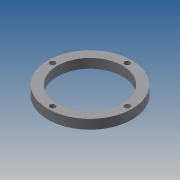
# Autodesk Inventor part: ring
Saved by Autodesk Inventor 2013 (Build 170138000, 138)
## iProperties
Created: 2017-03-30
Part Number: ring
Material: Generic
Document SubType Name: Modeling
Designer: employee
Density: 1 g/cm^3
Author: employee
Autodesk Inventor part; units mm, degrees
ref_plane "YZ Plane" through (0, 0, 0) normal (1, 0, 0) x (0, 1, 0)
ref_plane "XZ Plane" through (0, 0, 0) normal (0, 1, 0) x (-1, 0, 0)
ref_plane "XY Plane" through (0, 0, 0) normal (0, 0, 1) x (1, 0, 0)
sketch "Sketch1" plane through (0, 0, 0) normal (0, 0, 1) x (1, 0, 0)
  circle A0 centre (0, 0) radius 45
  circle A1 centre (0, 0) radius 35
  dimension "d0" = 70
  dimension "d2" = 90
  constraints: 2 centre point, 1 coincident
  measures "d0" diameter of A1
  measures "d2" diameter of A0
extrude "Extrusion1" add sketch "Sketch1" along normal blind 10
sketch "Sketch2" plane through (0, 0, 10) normal (0, 0, 1) x (1, 0, 0)
  circle A0 centre (0, 0) radius 35 projected
  circle A1 centre (0, 40) radius 1.75
  dimension "d5" = 40
  dimension "d6" = 3.5
  constraints: 1 centre point, 1 vertical alignment
  measures "d5" distance of A1.centre A0.centre
  measures "d6" diameter of A1
extrude "Extrusion2" cut sketch "Sketch2" against normal through all contours A1
sketch "Sketch3" plane through (0, 0, 10) normal (0, 0, 1) x (1, 0, 0)
  circle A0 centre (0, 40) radius 1.75 projected
  line L0 (3.1754, 40) -> (1.5877, 37.25)
  line L1 (1.5877, 37.25) -> (-1.5877, 37.25)
  line L2 (-1.5877, 37.25) -> (-3.1754, 40)
  line L3 (-3.1754, 40) -> (-1.5877, 42.75)
  line L4 (-1.5877, 42.75) -> (1.5877, 42.75)
  line L5 (1.5877, 42.75) -> (3.1754, 40)
  point P0 (0, 42.75)
  dimension "d9" = 5.5
  constraints: 12 end point, 1 coincident, 1 horizontal alignment, 1 midpoint, 13 other
  measures "d9" distance from line of L1 point (0, 42.75)
extrude "Extrusion3" cut sketch "Sketch3" against normal blind 4
pattern_circular "Circular Pattern1" count 4 over 360 about axis through (0, 0, 0) along (0, 0, 1) of "Extrusion3", "Extrusion2"
body "Solid1"
